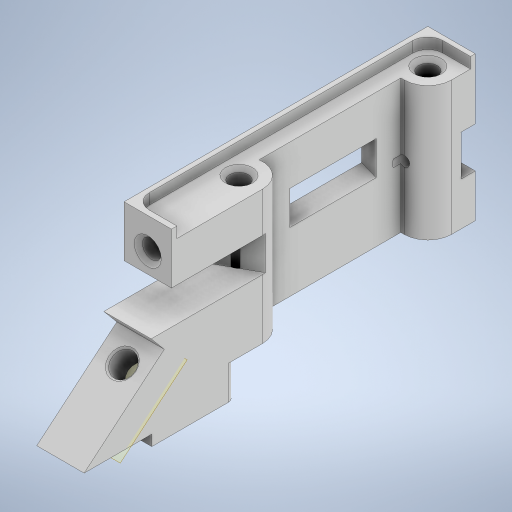
# Autodesk Inventor part: ściana
Saved by Autodesk Inventor 2023 (Build 270158000, 158)
## iProperties
Created: 2025-01-11
Part Number: ściana
Material: Ogólny
Document SubType Name: Modeling
Designer: kamil
Density: 1 g/cm^3
Appearance: Domyślna
Author: kamil
Autodesk Inventor part; units mm, degrees
ref_plane "YZ Plane" through (0, 0, 0) normal (1, 0, 0) x (0, 1, 0)
ref_plane "XZ Plane" through (0, 0, 0) normal (0, 1, 0) x (-1, 0, 0)
sketch "Szkic1" plane through (0, 0, 0) normal (1, 0, 0) x (0, 1, 0)
  line L0 (0, 0) -> (10, 0)
  line L1 (10, 0) -> (10, -55)
  line L2 (10, -55) -> (0, -55)
  line L3 (0, -55) -> (0, 0)
  dimension "d0" = 10
  dimension "d1" = 55
  constraints: 8 end point, 2 parallel, 1 horizontal, 1 perpendicular
  measures "d0" distance of L1.end L2.end
  measures "d1" distance of L0.end L1.end
extrude "Wyciągnięcie proste1" add sketch "Szkic1" along normal blind 7
sketch "Szkic2" plane through (0, 0, 0) normal (-1, 0, 0) x (0, 0, 1)
  line L0 (7.3328, -6.25) -> (12, -6.25) projected
  line L1 (12, -6.25) -> (-7.1511, 9.8197) projected
  line L2 (-7.1511, 9.8197) -> (-9.0795, 7.5216) projected
  line L3 (7.3328, -6.25) -> (-9.0795, 7.5216) projected
  line L4 (-55, 0) -> (-55, 10) projected
  line L5 (0, 0) -> (-55, 0) projected
  line L6 (0, 10) -> (0, 0) projected
  line L7 (-55, 10) -> (0, 10) projected
  line L8 (-7.1511, 9.8197) -> (-7.1511, 12.4768)
  point P0 (-7.1511, 10)
  point P1 (-0.1156, 0)
  constraints: 2 end point, 1 vertical
extrude "Wyciągnięcie proste2" cut sketch "Szkic2" against normal blind 10 contours L3 L2 L1 L6 L5 | L1 L8 L7 L6
sketch "Szkic3" plane through (0, 7.5216, -9.0795) normal (0, 0.7660444, 0.6427876) x (1, 0, 0)
  circle A0 centre (3.5, -3.5) radius 1.6 projected
  point P0 (0, -11.79)
hole "Otwór1" at (3.5, 5.2718, -6.3983) direction (0, -0.7660444, -0.6427876) diameter 3.5 end through all countersink diameter 4 countersink angle 90
ref_plane "Płaszczyzna konstrukcyjna1" through (0, 4.4574, -11.6506) normal (0, 0.7660444, 0.6427876) x (1, 0, 0)
sketch "Szkic5" plane through (0, 0, 0) normal (-1, 0, 0) x (0, 0, 1)
  line L0 (-0.1156, 0) -> (-9.0795, 7.5216) projected
  line L1 (-9.0795, 7.5216) -> (-7.1511, 9.8197) projected
  line L2 (-7.1511, 9.8197) -> (-7.1511, 10) projected
  line L3 (-55, 10) -> (-7.1511, 10) projected
  line L4 (-55, 0) -> (-55, 10) projected
  line L5 (-0.1156, 0) -> (-55, 0) projected
  line L6 (-0.1156, 0) -> (3.4596, -3)
  line L7 (-20.1156, 0) -> (-20.1156, -3)
  line L8 (-20.1156, -3) -> (3.4596, -3)
  point P0 (0, 0)
  dimension "d17" = 20
  dimension "d18" = 3
  dimension "d19" = 40
  constraints: 6 end point, 1 horizontal, 1 point on line, 1 vertical
  measures "d17" distance of L7.start L0.start
  measures "d18" distance between parallel lines of L8 L5
  measures "d19" angle of L8 L6
extrude "Wyciągnięcie proste4" add sketch "Szkic5" against normal up to surface (7 mm away) contours L6 L8 L7 L5
sketch "Szkic4" plane through (0, 4.4574, -11.6506) normal (0, 0.7660444, 0.6427876) x (1, 0, 0)
  circle A0 centre (3.5, -3.5) radius 1.75 projected
  circle A1 centre (3.5, -3.5) radius 2.9
  line L0 (6.4, -5.1743) -> (3.5, -6.8486)
  line L1 (3.5, -6.8486) -> (0.6, -5.1743)
  line L2 (0.6, -5.1743) -> (0.6, -1.8257)
  line L3 (0.6, -1.8257) -> (3.5, -0.1514)
  line L4 (3.5, -0.1514) -> (6.4, -1.8257)
  line L5 (6.4, -1.8257) -> (6.4, -5.1743)
  point P0 (0, -11.79)
  point P1 (6.4, -3.5)
  dimension "d14" = 5.8
  constraints: 12 end point, 2 coincident, 1 horizontal alignment, 1 midpoint, 15 other
extrude "Wyciągnięcie proste3" cut sketch "Szkic4" against normal through all contours A0 | A1 | L5 L0 A1 | A1 L4 L5 | A1 L3 L4 | L0 L1 A1 | A1 L2 L3 | L1 L2 A1
sketch "Szkic6" plane through (0, 0, 0) normal (-1, 0, 0) x (0, 0, 1)
  line L0 (-6.4043, 0.0552) -> (-8.9679, -3) projected
  line L1 (-6.4043, 0.0552) -> (-3.9233, 3.0118)
  line L2 (3.4596, -3) -> (-9.0795, 7.5216) projected
  line L3 (4.2983, -3) -> (-6.3199, -3)
  line L4 (-6.3199, -3) -> (-6.3199, -1.4)
  line L5 (-6.3199, -1.4) -> (4.2983, -1.4)
  line L6 (4.2983, -1.4) -> (4.2983, -3)
  line L7 (-20.1156, -3) -> (3.4596, -3) projected
  line L8 (-8.899, -4.4737) -> (-6.014, -1.0355)
  line L9 (-6.014, -1.0355) -> (-3.1573, 2.369)
  point P0 (0, 0)
  point P1 (1.5528, -1.4)
  dimension "d22" = 1.6
  dimension "d23" = 1
  constraints: 14 end point, 2 parallel, 1 collinear, 1 horizontal, 1 perpendicular, 1 point on line, 1 other
  measures "d22" distance of L3.end L4.end
  measures "d23" distance between parallel lines of L0 L8
extrude "Wyciągnięcie proste5" cut sketch "Szkic6" against normal through all contours L3 L4 L5 L2
sketch "Szkic7" plane through (0, 10, -55) normal (0, 1, 0) x (1, 0, 0)
  line L0 (0, -47.8489) -> (7, -47.8489) projected
  line L1 (7, 0) -> (7, -47.8489) projected
  line L2 (0, 0) -> (7, 0) projected
  line L3 (0, 0) -> (0, -47.8489) projected
  circle A0 centre (3.5, -3.5) radius 3.5
  line L4 (0, -34.8844) -> (7, -34.8844) projected
  circle A1 centre (3.5, -31.3844) radius 3.5
  line L5 (3, -27.8844) -> (7, -27.8844)
  line L6 (7, -27.8844) -> (7, -7)
  line L7 (7, -7) -> (3, -7)
  line L8 (3, -7) -> (3, -27.8844)
  point P0 (0, -55)
  point P1 (3.5, 0)
  point P2 (7, -3.5)
  point P3 (3.5, -7)
  point P4 (3.5, -27.8844)
  point P5 (7, -31.3844)
  dimension "d26" = 7
  dimension "d27" = 3.5
  dimension "d28" = 7
  dimension "d29" = 3.5
  dimension "d30" = 4
  constraints: 8 end point, 2 centre point, 2 parallel, 2 tangent, 2 vertical alignment, 1 horizontal, 1 midpoint, 1 perpendicular, 1 point on line
  measures "d26" diameter of A0
  measures "d27" distance from line of A0.centre L2
  measures "d28" diameter of A1
  measures "d29" distance from line of L4 A1.centre
  measures "d30" distance between parallel lines of L1 L8
extrude "Wyciągnięcie proste6" cut sketch "Szkic7" against normal through all contours A1 L5 L1 | L5 L8 L7 L1 | A0 L1 L7
sketch "Szkic9" plane through (0, 10, -55) normal (0, 1, 0) x (1, 0, 0)
  arc A0 (7, -31.3844) -> (3.5, -27.8844) centre (3.5, -31.3844) ccw projected
  line L0 (3.5, -27.8844) -> (3, -27.8844) projected
  line L1 (3, -27.8844) -> (3, -7) projected
  line L2 (3, -7) -> (3.5, -7) projected
  arc A1 (3.5, -7) -> (7, -3.5) centre (3.5, -3.5) ccw projected
  line L3 (7, 0) -> (7, -3.5) projected
  line L4 (0, 0) -> (7, 0) projected
  line L5 (0, 0) -> (0, -47.8489) projected
  line L6 (0, -47.8489) -> (7, -47.8489) projected
  line L7 (7, -31.3844) -> (7, -47.8489) projected
  line L8 (3, -7) -> (3, 0)
  line L9 (3, -27.8844) -> (3, -47.8489)
  point P0 (0, -55)
  constraints: 4 end point, 3 point on line, 1 vertical
extrude "Wyciągnięcie proste7" add sketch "Szkic9" along normal blind 10.75 contours L9 L6 L5 L4 L8 L1
sketch "Szkic10" plane through (0, 9.8197, -7.1511) normal (0, 0, 1) x (1, 0, 0)
  line L0 (7, 0.1803) -> (7, 0) projected
  line L1 (3, 0.1803) -> (7, 0.1803) projected
  line L2 (3, 0.1803) -> (3, 10.9303) projected
  line L3 (0, 10.9303) -> (3, 10.9303) projected
  line L4 (0, 0) -> (0, 10.9303) projected
  line L5 (0, 0) -> (7, 0) projected
  line L6 (0, -9.8197) -> (0, 10.9303) projected
  line L7 (0, 10.9303) -> (7, 10.9303)
  line L8 (7, 10.9303) -> (7, 0.1803)
  line L9 (7, 0.1803) -> (0, 0.1803)
  line L10 (0, 0.1803) -> (0, 10.9303)
  constraints: 8 end point, 2 parallel, 1 horizontal, 1 perpendicular
extrude "Wyciągnięcie proste8" cut sketch "Szkic10" against normal blind 3 contours L0 L5 L4 L9 L1 | L9 L4 L3 L2
sketch "Szkic11" plane through (3, 10, -55) normal (0, 1, 0) x (1, 0, 0)
  line L0 (0, 0) -> (0, -7) projected
  line L1 (0, -7) -> (0.5, -7) projected
  arc A0 (0.5, -7) -> (4, -3.5) centre (0.5, -3.5) ccw projected
  line L2 (4, 0) -> (4, -3.5) projected
  line L3 (0, 0) -> (4, 0) projected
  line L4 (0, -44.8489) -> (4, -44.8489) projected
  line L5 (4, -31.3844) -> (4, -44.8489) projected
  arc A1 (4, -31.3844) -> (0.5, -27.8844) centre (0.5, -31.3844) ccw projected
  line L6 (0.5, -27.8844) -> (0, -27.8844) projected
  line L7 (0, -27.8844) -> (0, -44.8489) projected
  circle A2 centre (0.5, -31.3844) radius 3.5
  line L8 (4, -34.8844) -> (-3, -34.8844) projected
  line L9 (0.5, -34.8844) -> (4, -34.8844)
  line L10 (4, -34.8844) -> (4, -31.3844)
  line L11 (4, -31.3844) -> (0.5, -31.3844)
  line L12 (0.5, -31.3844) -> (0.5, -34.8844)
  line L13 (-3, -34.8844) -> (-3, -48.6801) projected
  line L14 (0.5, -31.3844) -> (-3, -31.3844)
  line L15 (-3, -31.3844) -> (-3, -34.8844)
  line L16 (-3, -34.8844) -> (0.5, -34.8844)
  line L17 (0.5, -34.8844) -> (0.5, -31.3844)
  point P0 (-3, -55)
  point P1 (0.5, -34.8844)
  point P2 (0.5, -27.8844)
  constraints: 16 end point, 4 parallel, 2 horizontal, 2 perpendicular, 1 coincident, 1 midpoint, 1 point on line, 4 other
extrude "Wyciągnięcie proste9" add sketch "Szkic11" along normal up to surface (10.75 mm away) contours L3 L2 A0 L1 L0 | L8 A2 L5 | A2 L14 L7 | L7 L14 L12 A2 | L12 L11 A2 | L11 L14 L7 A2 A1 | L14 A2 L7
sketch "Szkic12" plane through (7, 0, -55) normal (0, 0, -1) x (-1, 0, 0)
  arc A0 (3.5, 6.875) -> (-24.5, 13.875) centre (3.5, 10.375) ccw projected
  line L0 (-24.5, 13.875) -> (0, 13.875) projected
  line L1 (0, 6.875) -> (3.5, 6.875) projected
  line L2 (-86, 7.575) -> (-86, 0) projected
  line L3 (-86, 0) -> (0, 0) projected
  line L4 (0, 0) -> (0, 7.575) projected
  line L5 (0, 0) -> (0, 20.75) projected
  line L6 (-93, 0) -> (-93, 20.75) projected
  line L7 (-93, 0) -> (-86, 0) projected
  line L8 (-86, 0) -> (-86, 7.375) projected
  line L9 (-93, 20.75) -> (-86, 20.75) projected
  line L10 (-85.5, 0) -> (-85.5, 7.375)
  line L11 (-85.5, 7.375) -> (-89.5, 7.375)
  arc A1 (-89.5, 13.375) -> (-89.5, 7.375) centre (-89.5, 10.375) ccw
  line L12 (-89.5, 13.375) -> (-85.5, 13.375)
  line L13 (-85.5, 13.375) -> (-85.5, 20.75)
  line L14 (3.5, 13.375) -> (0, 13.375)
  line L15 (0, 7.375) -> (3.5, 7.375)
  arc A2 (3.5, 7.375) -> (3.5, 13.375) centre (3.5, 10.375) ccw
  line L16 (0, 7.575) -> (3.5, 7.575) projected
  arc A3 (3.5, 7.575) -> (3.5, 13.175) centre (3.5, 10.375) ccw projected
  line L17 (3.5, 13.175) -> (0, 13.175) projected
  line L18 (-61.5, 5) -> (-61.5, 17.75) projected
  line L19 (-24.5, 17.75) -> (-24.5, 5) projected
  line L20 (-24.5, 5) -> (-61.5, 5) projected
  line L21 (0, 13.175) -> (0, 20.75) projected
  line L22 (-86, 13.175) -> (-89.5, 13.175) projected
  arc A4 (-89.5, 13.175) -> (-89.5, 7.575) centre (-89.5, 10.375) ccw projected
  line L23 (-89.5, 7.575) -> (-86, 7.575) projected
  line L24 (-61.5, 17.75) -> (-24.5, 17.75) projected
  line L25 (0, 20.75) -> (-86, 20.75) projected
  line L26 (-86, 20.75) -> (-86, 13.175) projected
  circle A5 centre (-89.5, 10.375) radius 2.5 projected
  circle A6 centre (3.5, 10.375) radius 2.5 projected
  line L27 (-89.5, 7.375) -> (-86, 7.375) projected
  arc A7 (-89.5, 13.375) -> (-89.5, 7.375) centre (-89.5, 10.375) ccw projected
  line L28 (-86, 13.375) -> (-89.5, 13.375) projected
  line L29 (-86, 13.375) -> (-86, 20.75) projected
  point P0 (7, 0)
  point P1 (-86, 6.875)
  point P2 (0, 10)
  point P3 (-86, 13.875)
  point P4 (-86, 7.375)
  point P5 (-86, 13.375)
  point P6 (3.5, 7.375)
  point P7 (0, 13.375)
  point P8 (0, 7.375)
  point P9 (0, 7.375)
  point P10 (-86, 13.375)
  point P11 (-86, 7.375)
  point P12 (1.6972, 13.375)
  point P13 (1.4, 13.175)
  point P14 (-86, 13.375)
  dimension "d40" = 0.5
  dimension "d41" = 0.5
  dimension "d42" = 0.5
  constraints: 12 end point, 4 point on circle, 2 centre point, 2 parallel, 1 other
  measures "d40" distance between parallel lines of L0 L14
  measures "d41" distance between parallel lines of L1 L15
extrude "Wyciągnięcie proste10" cut sketch "Szkic12" against normal blind 2.1 contours A2 L15 L4 L16 A3 A0 | A0 A3 A2 | A3 L16 L5 L17 A0 A6 | A0 A6 A3 | A0 A3 L17 L5 L14 A2 | A6 A0 | A0 A6 | L3 L2 L11 L10
sketch "Szkic13" plane through (0, 9.8197, -7.1511) normal (0, 1, 0) x (1, 0, 0)
  line L0 (4.1, 33.0489) -> (4.1, 28.6489) projected
  line L1 (4.1, 33.0489) -> (3, 33.0489) projected
  line L2 (4.1, 28.6489) -> (3, 28.6489) projected
  line L3 (12.8887, 11.1113) -> (16, 8) projected
  line L4 (12.8887, 11.1113) -> (12.1109, 10.3335) projected
  line L5 (16, 8) -> (15.2222, 7.2222) projected
  line L6 (3.5622, 24.6489) -> (-384.2285, -86.5483)
  arc A0 (-384.2285, 148.2461) -> (-384.2285, -86.5483) centre (10.6723, 30.8489) ccw
  line L7 (-384.2285, 148.2461) -> (3.5622, 37.0489)
  line L8 (3.5622, 37.0489) -> (8.1, 37.0489)
  line L9 (8.1, 37.0489) -> (8.1, 24.6489)
  line L10 (8.1, 24.6489) -> (3.5622, 24.6489)
  line L11 (-343.1577, -182.0217) -> (9.68, 13.5594)
  line L12 (9.68, 13.5594) -> (12.8887, 16.7681)
  line L13 (12.8887, 16.7681) -> (21.6569, 8)
  line L14 (21.6569, 8) -> (18.4481, 4.7913)
  line L15 (18.4481, 4.7913) -> (-177.133, -348.0464)
  arc A1 (-343.1577, -182.0217) -> (-177.133, -348.0464) centre (19.0917, 14.203) ccw
  line L16 (3, 28.6489) -> (3, 33.0489) projected
  line L17 (15.2222, 7.2222) -> (12.1109, 10.3335) projected
  point P0 (0, -7.1511)
  constraints: 20 end point, 4 point on circle, 2 centre point, 4 other
extrude "Wyciągnięcie proste11" cut sketch "Szkic13" along normal blind 5 contours L0 L2 L16 L1 | L3 L5 L17 L4 | L6 A0 L7 L8 L9 L10 | L11 L12 L13 L14 L15 A1
sketch "Szkic14" plane through (3.5, 10, -20.1156) normal (0, 1, 0) x (1, 0, 0)
  line L0 (-0.5, -3.1079) -> (3.5, -0.8907) projected
  line L1 (3.5, 0) -> (3.5, -0.8907) projected
  line L2 (3.5, 0) -> (0, 0) projected
  arc A0 (-0.5, 0.0359) -> (0, 0) centre (0, 3.5) ccw projected
  line L3 (-0.5, 0.0359) -> (-0.5, -3.1079) projected
  point P0 (-3.5, -20.1156)
extrude "Wyciągnięcie proste12" add sketch "Szkic14" along normal up to surface (10.75 mm away)
sketch "Szkic15" plane through (0, 20.75, -55) normal (0, 1, 0) x (1, 0, 0)
  line L0 (0, 0) -> (0, -44.8489) projected
  line L1 (0, -44.8489) -> (3, -44.8489) projected
  line L2 (3, -44.8489) -> (3, -37.9923) projected
  line L3 (7, -35.775) -> (3, -37.9923) projected
  line L4 (7, -31.3844) -> (7, -35.775) projected
  arc A0 (7, -31.3844) -> (3, -27.9203) centre (3.5, -31.3844) ccw projected
  line L5 (3, -27.9203) -> (3, -7) projected
  line L6 (3.5, -7) -> (3, -7) projected
  arc A1 (3.5, -7) -> (7, -3.5) centre (3.5, -3.5) ccw projected
  line L7 (7, 0) -> (7, -3.5) projected
  line L8 (0, 0) -> (7, 0) projected
  line L9 (0, -44.8489) -> (7, -44.8489)
  line L10 (7, -44.8489) -> (7, -35.775)
  line L11 (7, -35.775) -> (0, -35.775)
  line L12 (0, -35.775) -> (0, -44.8489)
  point P0 (0, -55)
  constraints: 8 end point, 2 parallel, 1 horizontal, 1 perpendicular
extrude "Wyciągnięcie proste13" add sketch "Szkic15" against normal up to surface (5.9303 mm away) contours L10 L9 L2 L3
sketch "Szkic16" plane through (0, -3, -20.1156) normal (0, -1, 0) x (1, 0, 0)
  line L0 (7, 13.7957) -> (0, 13.7957) projected
  line L1 (0, 0) -> (0, 13.7957) projected
  line L2 (0, 0) -> (7, 0) projected
  line L3 (7, 0) -> (7, 13.7957) projected
  line L4 (6.4, 4.5908) -> (3.5, 2.4051) projected
  line L5 (3.5, 2.4051) -> (0.6, 4.5908) projected
  line L6 (0.6, 4.5908) -> (0.6, 8.9621) projected
  line L7 (0.6, 8.9621) -> (3.5, 11.1478) projected
  line L8 (3.5, 11.1478) -> (6.4, 8.9621) projected
  line L9 (6.4, 8.9621) -> (6.4, 4.5908) projected
  point P0 (0, 20.1156)
extrude "Wyciągnięcie proste14" add sketch "Szkic16" along normal blind 1
sketch "Szkic17" plane through (7, 0, 0) normal (1, 0, 0) x (0, 0, -1)
  line L0 (6.3199, -1.4) -> (6.3199, -4) projected
  line L1 (20.1156, -4) -> (6.3199, -4) projected
  line L2 (6.3199, -1.4) -> (7.2337, -1.4)
  line L3 (7.2337, -1.4) -> (7.2337, -4)
  line L4 (7.2337, -4) -> (6.3199, -4)
  line L5 (6.3199, -4) -> (6.3199, -1.4)
  line L6 (6.4043, 0.0552) -> (8.9679, -3) projected
  line L7 (8.9679, -3) -> (8.9679, -4) projected
  point P0 (0, 0)
  dimension "d55" = 0.3
  constraints: 8 end point, 2 parallel, 1 horizontal, 1 perpendicular, 1 point on line
  measures "d55" distance from line of L6 L2.end
extrude "Wyciągnięcie proste15" cut sketch "Szkic17" against normal through all
chamfer "Faza1" distance 1 angle 45 2 edges at (2.05, -4, -16.6177) (4.95, -4, -16.6177)
sketch "Szkic18" plane through (7, 0, 0) normal (1, 0, 0) x (0, 0, -1)
  line L0 (-1.5528, -1.4) -> (7.2337, -1.4) projected
  line L1 (7.2337, -1.4) -> (7.2337, -4) projected
  line L2 (20.1156, -4) -> (7.2337, -4) projected
  line L3 (20.1156, 0) -> (20.1156, -4) projected
  line L4 (20.1156, 0) -> (23.6156, 0) projected
  line L5 (23.6156, 0) -> (23.6156, 20.75) projected
  line L6 (23.6156, 20.75) -> (10.1511, 20.75) projected
  line L7 (10.1511, 20.75) -> (10.1511, 14.8197) projected
  line L8 (19.225, 14.8197) -> (10.1511, 14.8197) projected
  line L9 (19.225, 14.8197) -> (19.225, 9.8197) projected
  line L10 (19.225, 9.8197) -> (7.1511, 9.8197) projected
  line L11 (7.1511, 9.8197) -> (9.0795, 7.5216) projected
  line L12 (-1.5528, -1.4) -> (9.0795, 7.5216) projected
  line L13 (-1.5528, -1.4) -> (-2.7446, -2.4)
  line L14 (-2.7446, -2.4) -> (7.2337, -2.4)
  point P0 (0, 0)
  dimension "d61" = 1
  constraints: 4 end point, 1 collinear, 1 horizontal, 1 point on line
  measures "d61" distance between parallel lines of L14 L0
extrude "Wyciągnięcie proste16" add sketch "Szkic18" against normal up to surface (7 mm away) contours L0 L1 L14 L13
sketch "Szkic19" plane through (0, 9.8197, -10.1511) normal (0, 0, 1) x (1, 0, 0)
  line L0 (0, 5) -> (7, 5) projected
  line L1 (7, 10.9303) -> (7, 5) projected
  line L2 (0, 10.9303) -> (7, 10.9303) projected
  line L3 (0, 5) -> (0, 10.9303) projected
  point P0 (0, -9.8197)
  point P1 (3.5, 7.9652)
  point P2 (3.5, 10.9303)
  point P3 (0, 7.9652)
  constraints: 2 midpoint, 1 horizontal alignment, 1 vertical alignment
hole "Otwór2" at (3.5, 17.7848, -10.1511) direction (0, 0, -1) diameter 2.8 depth 10 tip angle 118 countersink diameter 4 countersink angle 90
sketch "Szkic20" plane through (0, 0, -55) normal (0, -1, 0) x (1, 0, 0)
  arc A0 (7, 3.5) -> (3.5, 7) centre (3.5, 3.5) ccw projected
  arc A1 (3.5, 27.8844) -> (7, 31.3844) centre (3.5, 31.3844) ccw projected
  point P0 (0, 55)
hole "Otwór3" at (3.5, 0, -51.5) at (3.5, 0, -23.6156) direction (0, 1, 0) diameter 2.8 end through all countersink diameter 4 countersink angle 90
chamfer "Faza2" distance 0.6 angle 45 2 edges at (3.5, 20.75, -50.1) (3.5, 20.75, -22.2156)
sketch "Szkic21" plane through (7, -2.4, -7.2337) normal (0, -1, 0) x (1, 0, 0)
  line L0 (0, 0) -> (-7, 0) projected
  point P0 (-7, 7.2337)
  point P1 (-3.1444, 3)
  point P2 (-3.5, 0)
  dimension "d81" = 3
  constraints: 1 midpoint
  measures "d81" vertical distance of point (-3.5, 0) point (-3.144, 3)
hole "Otwór4" at (3.8556, -2.4, -4.2337) direction (0, 1, 0) diameter 1.5 depth 5 tip angle 118 countersink diameter 2.2 countersink angle 90
sketch "Szkic22" plane through (7, 0, -52.9) normal (0, 0, -1) x (-1, 0, 0)
  line L0 (0, 13.375) -> (3.5, 13.375) projected
  line L1 (3.5, 7.375) -> (0, 7.375) projected
  arc A0 (3.5, 7.375) -> (3.5, 13.375) centre (3.5, 10.375) ccw projected
  arc A1 (3.5, 7.375) -> (3.5, 13.375) centre (3.5, 10.375) ccw projected
  line L2 (3.5, 13.375) -> (3.5, 7.375) projected
  line L3 (0, 7.375) -> (0, 13.375) projected
  point P0 (7, 0)
  constraints: 1 coincident
hole "Otwór5" at (3.5, 10.375, -52.9) direction (0, 0, 1) diameter 1.5 depth 6 tip angle 118 countersink diameter 2 countersink angle 90
sketch "Szkic23" plane through (0, -4, -20.1156) normal (0, -1, 0) x (1, 0, 0)
  line L0 (6, 0.5753) -> (1, 0.5753) projected
  arc A0 (1, 0.5753) -> (0, -0.4247) centre (1, -0.4247) ccw projected
  line L1 (0, -0.4247) -> (0, -34.4247) projected
  arc A1 (6, 0.5753) -> (7, 1.5753) centre (6, 1.5753) ccw projected
  line L2 (7, 0) -> (7, 12.882) projected
  arc A2 (8, 12.5753) -> (7, 11.5753) centre (8, 11.5753) ccw projected
  line L3 (0.6, 3.3386) -> (0.6, 8.9621) projected
  line L4 (0.6, 8.9621) -> (3.5, 11.1478) projected
  line L5 (3.5, 11.1478) -> (6.4, 8.9621) projected
  line L6 (6.4, 8.9621) -> (6.4, 3.3386) projected
  line L7 (3.5, 1.1529) -> (6.4, 3.3386) projected
  line L8 (0.6, 3.3386) -> (3.5, 1.1529) projected
  line L9 (7, 12.882) -> (0, 12.882) projected
  line L10 (0, 12.882) -> (0, 0) projected
  line L11 (0, 0) -> (7, 0) projected
  line L12 (7, 0) -> (7, 12.882) projected
  line L13 (1, 0.5753) -> (0, 0.5753)
  point P0 (0, 20.1156)
  constraints: 2 end point, 1 perpendicular, 1 point on line, 1 tangent
extrude "Wyciągnięcie proste17" cut sketch "Szkic23" against normal up to surface (4 mm away) contours A1 L2 L11 A0 L0 | A0 L11 L10 L13
sketch "Szkic24" plane through (0, 9.8197, -7.1511) normal (0, 1, 0) x (1, 0, 0)
  line L0 (0, 3) -> (7, 3) projected
  line L1 (0, 0) -> (7, 0) projected
  line L2 (7, 12.0738) -> (7, 0) projected
  line L3 (7, 12.0738) -> (0, 8.1937) projected
  line L4 (0, 0) -> (0, 8.1937) projected
  point P0 (0, -7.1511)
extrude "Wyciągnięcie proste18" add sketch "Szkic24" along normal up to surface (5 mm away) contours L4 L3 L2 L0
sketch "Szkic25" plane through (0, 9.8197, -10.1511) normal (0, 1, 0) x (1, 0, 0)
  line L0 (1.7071, 10.9722) -> (-53.1556, -19.4387) projected
  line L1 (4.7071, 12.6351) -> (26.1715, 24.533) projected
  line L2 (-53.1556, -19.4387) -> (26.1715, 24.533)
  line L3 (9.9008, -4.8201) -> (-17.8002, -54.794) projected
  line L4 (26.1715, -26.0876) -> (-24.6917, -26.0876)
  line L5 (-24.6917, -26.0876) -> (-24.6917, 22.7519)
  line L6 (-24.6917, 22.7519) -> (26.1715, 22.7519)
  line L7 (26.1715, 22.7519) -> (26.1715, -26.0876)
  point P0 (0, -10.1511)
  point P1 (22.9583, 22.7519)
  point P2 (-24.6917, -3.6609)
  constraints: 10 end point, 2 parallel, 1 horizontal, 1 perpendicular
ref_plane "Płaszczyzna konstrukcyjna2" through (27.7486, 14.8197, -10.1511) normal (0, -1, 0) x (1, 0, 0)
extrude "Wyciągnięcie proste19" cut sketch "Szkic25" along normal up to surface (5 mm away) contours L2 L1 L6 L7 L4 L5 L0
sketch "Szkic26" plane through (0, 20.75, -55) normal (0, 1, 0) x (1, 0, 0)
  circle A0 centre (3.5, -3.5) radius 2 projected
  line L0 (0, 0) -> (0, -44.8489) projected
  line L1 (0, -44.8489) -> (7, -44.8489) projected
  line L2 (7, -31.3844) -> (7, -44.8489) projected
  arc A1 (7, -31.3844) -> (3, -27.9203) centre (3.5, -31.3844) ccw projected
  line L3 (3, -27.9203) -> (3, -7) projected
  line L4 (3.5, -7) -> (3, -7) projected
  arc A2 (3.5, -7) -> (7, -3.5) centre (3.5, -3.5) ccw projected
  line L5 (7, 0) -> (7, -3.5) projected
  line L6 (0, 0) -> (7, 0) projected
  circle A3 centre (3.5, -31.3844) radius 2 projected
  arc A4 (2.9, -0.9) -> (0.9, -2.9) centre (2.9, -2.9) ccw projected
  line L7 (2.9, -0.9) -> (29.9, -0.9) projected
  line L8 (0.9, -41.8489) -> (0.9, -2.9) projected
  arc A5 (0.9, -41.8489) -> (2.9, -43.8489) centre (2.9, -41.8489) ccw projected
  line L9 (2.8995, -43.8503) -> (22.79, -43.8503) projected
  arc A6 (0.7, -41.8489) -> (2.9, -44.0489) centre (2.9, -41.8489) ccw
  line L10 (0.7, -41.8489) -> (0.7, -2.9)
  arc A7 (2.9, -0.7) -> (0.7, -2.9) centre (2.9, -2.9) ccw
  line L11 (2.9, -0.7) -> (29.9, -0.7)
  line L12 (-7.5113, -15.9778) -> (8.4005, -17.8433)
  line L13 (10.9663, -10.9506) -> (-3.8693, 3.5292)
  line L14 (-7.5113, -38.9662) -> (19.1023, -23.8542)
  line L15 (-6.7995, -43.4045) -> (5.7439, -40.5034)
  line L16 (0, -44.8489) -> (7, -44.8489) projected
  line L17 (7, -44.8489) -> (7, -43.8503)
  line L18 (7, -31.3844) -> (7, -44.8489) projected
  line L19 (2.9, -44.0489) -> (7, -44.0489)
  point P0 (0, -55)
  point P1 (7, -0.7)
  dimension "d102" = 0.2
  dimension "d104" = 0.1986
  constraints: 16 end point, 4 point on circle, 3 point on line, 2 centre point, 1 parallel, 3 other
  measures "d102" radial gap between concentric circles of A5 A6
  measures "d104" distance between parallel lines of L19 L9
extrude "Wyciągnięcie proste20" add sketch "Szkic26" along normal blind 1.6 contours L13 L0 L6 L5 L11 A7 | A7 L10 L12 L0 L13 | L10 L14 L0 L12 | L10 L15 L0 L14 | L10 A6 L19 L2 L1 L0 L15
sketch "Szkic27" plane through (0, 0, -55) normal (0, -1, 0) x (1, 0, 0)
  circle A0 centre (3.5, 3.5) radius 2 projected
  circle A1 centre (3.5, 31.3844) radius 2 projected
  arc A2 (3.5, 27.8844) -> (7, 31.3844) centre (3.5, 31.3844) ccw projected
  line L0 (7, 36.4596) -> (7, 31.3844) projected
  arc A3 (6, 35.4596) -> (7, 36.4596) centre (6, 36.4596) ccw projected
  line L1 (0, 35.4596) -> (6, 35.4596) projected
  line L2 (0, 35.4596) -> (0, 0) projected
  line L3 (0, 0) -> (7, 0) projected
  line L4 (7, 3.5) -> (7, 0) projected
  arc A4 (7, 3.5) -> (3.5, 7) centre (3.5, 3.5) ccw projected
  line L5 (3.5, 7) -> (3, 7) projected
  line L6 (3, 7) -> (3, 27.8844) projected
  line L7 (3, 27.8844) -> (3.5, 27.8844) projected
  point P0 (0, 55)
extrude "Wyciągnięcie proste21" cut sketch "Szkic27" against normal blind 1 contours A0 | A1 | L7 L6 L5 A4 L4 L3 L2 L1 A3 L0 A2
chamfer "Faza3" distance 0.6 angle 45 2 edges at (3.5, 1, -22.2156) (3.5, 1, -50.1)
